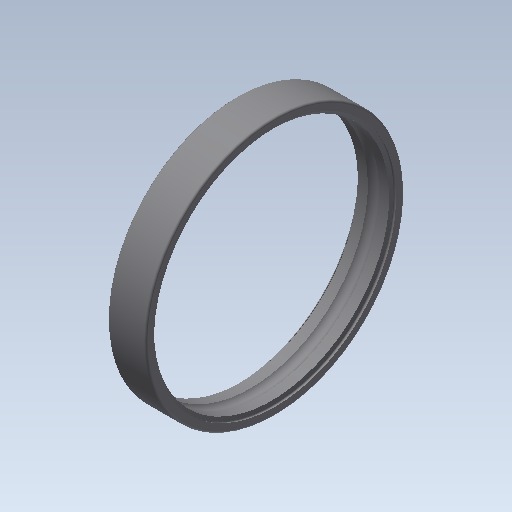
# Autodesk Inventor part: W 61704-2ZS_PART2
Saved by Autodesk Inventor 2021 (Build 250183000, 183)
## iProperties
Created: 2020-02-12
Part Number: W 61704-2ZS_PART2
Material: Allgemein
Catalog Web Link: www.cadenas.de
Description: -Deep groove ball bearings
Vendor: SKF
Document SubType Name: Modeling
Designer: psadmin
Manufacturer: SKF
Mass: 0.353754 g
Surface Area: 8.58068 cm^2
Volume: 0.353754 cm^3
Density: 1 g/cm^3
Appearance: PSOLRGB-175-175-175
Category: PARTsolutions
Company: SKF
PSOL_IDENT_0: {$CADENAS_DATA\23d-libs\skf\bearings_units_and_housings\ball_bearings\deep_groove_ball_bearings\bb1_
PSOL_IDENT_1: 001_101.prj},201 {VTYP=3D},{NB=W 61704-2ZS_PART2},{LINA=W 61704-2ZS_PART2},{NN=BB1_001_101_PART2},{N
PSOL_IDENT_2: OPRJ=TRUE},{DATE=19.12.2019 14:34:47},{GEOMDATE=18.12.2019 13:53:11},{VERSION=},{LINEID=15490},{WBVA
PSOL_IDENT_3: R=},{WBNUMERIC=}  {NB=W 61704-2ZS_PART2},{LINA=W 61704-2ZS_PART2},{KT=DUMMY},{PRODUCTID=},{DESIGNATI
PSOL_IDENT_4: ON=W 61704-2ZS},{DD=20.000},{D=27.000},{B=4.000},{C=0.000},{DD1=22.36},{DD2=0.00},{D1=0.00},{D2=25.3
PSOL_IDENT_5: 0},{D3=0.000},{D4=0.000},{HH=MIN},{BB=0.000},{FF=0.00},{R0MAX=MIN},{R0=MIN},{R12=0.20},{PITCH=23.50}
PSOL_IDENT_6: ,{DW=1.588},{DDAMIN=21.500},{DDAMAX=22.000},{DDBMIN=MIN},{DDBMAX=MIN},{DBMIN=MIN},{DAMAX=26.000},{BB
PSOL_IDENT_7: AMIN=MIN},{CAMAX=MIN},{RAMAX=0.200},{LOAD1=0.585},{LOAD2=0.390},{LOAD3=0.017},{SPEED1=50000},{SPEED2=
PSOL_IDENT_8: 26000},{KR=0.015},{F0=8.700},{Z=18},{II=1},{MASS=0.006},{BEARING=W 61704-2ZS},{RING=},{HELP=1.218},{
PSOL_IDENT_9: HELP2=0.850},{DD1ALG=11.180},{YALG=11.180},{PITCH1=23.500},{DW1=1.588},{YALG1=12.282},{HALG1=1.218},
PSOL_IDENT_10: {SH=11.180},{CU=0.482},{DESIGN=dgbbw2z},{HALG=1.18},{B1=0},{SHIELDHELP=2}
NT: Deep groove ball bearings
NB: W 61704-2ZS_PART2
NBSYN: $DESIGNATION._PART2
LINA: W 61704-2ZS_PART2
SUPPLIER: SKF
ARTICLENO: W 61704-2ZS_PART2
BOMINFO: W 61704-2ZS_PART2
CREATOR: CADENAS GmbH
Title: W 61704-2ZS_PART2
Author: Cadenas PARTsolutions
Comments: Deep groove ball bearings
Autodesk Inventor part; units mm, degrees
ref_plane "YZ Plane" through (0, 0, 0) normal (1, 0, 0) x (0, 1, 0)
ref_plane "XZ Plane" through (0, 0, 0) normal (0, 1, 0) x (-1, 0, 0)
ref_plane "XY Plane" through (0, 0, 0) normal (0, 0, 1) x (1, 0, 0)
sketch "Sketch_17" plane through (0, 0, 0) normal (0, 0, 1) x (1, 0, 0)
  line L0 (50, 0) -> (-50, 0)
  line L1 (0, 13.3) -> (0, 12.65)
  line L2 (0, 12.65) -> (0.06, 12.65)
  arc A0 (0.3, 12.65) -> (0.06, 12.65) centre (0.18, 12.65) ccw
  line L3 (0.3, 12.65) -> (0.3649, 12.282)
  line L4 (0.3649, 12.282) -> (1.4106, 12.282)
  arc A1 (2.5894, 12.282) -> (1.4106, 12.282) centre (2, 11.75) ccw
  line L5 (2.5894, 12.282) -> (3.6351, 12.282)
  line L6 (3.6351, 12.282) -> (3.7, 12.65)
  arc A2 (3.94, 12.65) -> (3.7, 12.65) centre (3.82, 12.65) ccw
  line L7 (3.94, 12.65) -> (4, 12.65)
  line L8 (4, 12.65) -> (4, 13.3)
  arc A3 (4, 13.3) -> (3.8, 13.5) centre (3.8, 13.3) ccw
  line L9 (3.8, 13.5) -> (0.2, 13.5)
  arc A4 (0.2, 13.5) -> (0, 13.3) centre (0.2, 13.3) ccw
  constraints: 20 end point, 10 point on circle, 5 centre point
revolve "Revolution1" add sketch "Sketch_17" angle 360 about axis through (50, 0, 0) along (1, 0, 0)
body "Solid1"
